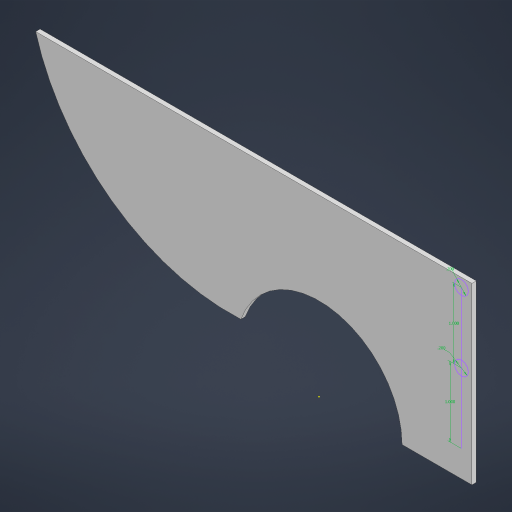
# Autodesk Inventor part: Horizontal climb
Saved by Autodesk Inventor 2023.4 (Build 274418000, 418)
## iProperties
Created: 2023-12-10
Part Number: Horizontal climb
Material: Generic
Document SubType Name: Modeling
Designer: diego
Density: 1 g/cm^3
Appearance: Default
Author: diego
Autodesk Inventor part; units mm, degrees
ref_plane "YZ Plane" through (0, 0, 0) normal (1, 0, 0) x (0, 1, 0)
ref_plane "XZ Plane" through (0, 0, 0) normal (0, 1, 0) x (-1, 0, 0)
ref_plane "XY Plane" through (0, 0, 0) normal (0, 0, 1) x (1, 0, 0)
sketch "Sketch1" plane through (0, 0, 0) normal (0, 0, 1) x (1, 0, 0)
  circle A0 centre (0, 0) radius 30.226
  line L0 (30.226, 0) -> (55.626, 0)
  line L1 (55.626, 0) -> (55.626, 63.5)
  line L2 (55.626, 63.5) -> (-103.124, 63.5)
  line L3 (-28.4673, 10.16) -> (-103.124, 10.16)
  line L4 (-103.124, 10.16) -> (-103.124, 63.5)
  arc A1 (-103.124, 63.5) -> (-28.4673, 10.16) centre (-32.2937, 83.7205) ccw
  point P0 (-36.1202, 10.16)
  dimension "d0" = 60.452
  dimension "d1" = 25.4
  dimension "d2" = 63.5
  dimension "d3" = 158.75
  dimension "d4" = 53.34
  dimension "d7" = 73.66
  constraints: 10 end point, 4 point on circle, 3 perpendicular, 2 centre point, 2 coincident, 1 horizontal, 1 parallel
  measures "d0" diameter of A0
  measures "d1" distance of L0.start L0.end
  measures "d2" distance of L0.end L1.end
  measures "d3" distance of L1.end L2.end
  measures "d4" distance of L3.end L2.end
  measures "d7" radius of A1
extrude "Extrusion1" add sketch "Sketch1" along normal blind 1.5875 contours A0 L3 A1 L2 L1 L0
sketch "Sketch2" plane through (0, 0, 1.5875) normal (0, 0, 1) x (1, 0, 0)
  circle A0 centre (51.7644, 60.3422) radius 2.54
  line L0 (51.7644, 60.3422) -> (51.7644, 34.9422)
  circle A1 centre (51.7644, 34.9422) radius 2.54
  line L1 (51.7644, 34.9422) -> (51.7644, 9.5422)
  point P0 (0, 0)
  dimension "d10" = 5.08
  dimension "d11" = 25.4
  dimension "d12" = 5.08
  dimension "d13" = 25.4
  constraints: 4 end point, 2 centre point, 2 vertical, 1 coincident
  measures "d10" diameter of A0
  measures "d11" distance of L0.start L0.end
  measures "d12" diameter of A1
  measures "d13" distance of L1.start L1.end
body "Solid1"
